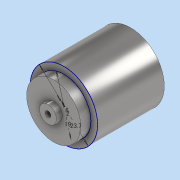
# Autodesk Inventor part: motor_for6speedgearbox
Saved by Autodesk Inventor 2022 (Build 260153000, 153)
## iProperties
Created: 2024-04-30
Part Number: motor_for6speedgearbox
Material: 鉄、可鍛鉄
Document SubType Name: Modeling
Designer: ktamu
Density: 7.15 g/cm^3
Appearance: 半つや出し
Author: ktamu
Autodesk Inventor part; units mm, degrees
ref_plane "YZ Plane" through (0, 0, 0) normal (1, 0, 0) x (0, 1, 0)
ref_plane "XZ Plane" through (0, 0, 0) normal (0, 1, 0) x (-1, 0, 0)
ref_plane "XY Plane" through (0, 0, 0) normal (0, 0, 1) x (1, 0, 0)
sketch "basescetch" plane through (0, 0, 0) normal (0, 0, 1) x (1, 0, 0)
  circle A0 centre (0, 0) radius 11.85
  circle A1 centre (0, 0) radius 9.5
  circle A2 centre (0, 0) radius 3
  circle A3 centre (0, 0) radius 1
  dimension "d0" = 23.7
  dimension "d1" = 19
  dimension "d2" = 6
  dimension "d3" = 2
  constraints: 4 centre point, 4 coincident
  measures "d0" diameter of A0
  measures "d1" diameter of A1
  measures "d2" diameter of A2
  measures "d3" diameter of A3
extrude "押し出し1" add sketch "basescetch" along normal blind 3.5 contours A1
extrude "押し出し2" add sketch "basescetch" along normal blind 5.5 contours A2
extrude "押し出し3" add sketch "basescetch" against normal blind 23.5 contours A0 | A1 | A2 | A3
sketch "スケッチ2" plane through (0, 0, -23.5) normal (0, 0, -1) x (-1, 0, 0)
  circle A0 centre (0, 0) radius 1 projected
  arc A1 (-2, 3.75) -> (2, 3.75) centre (0, 0) ccw
  line L0 (0, -4.25) -> (0, -1)
  line L1 (0, -4.25) -> (8, -4.25) construction
  line L2 (0, 3.75) -> (2, 3.75)
  line L3 (-2, 3.75) -> (0, 3.75)
  dimension "d10" = 8.5
  dimension "d11" = 8
  dimension "d12" = 90
  constraints: 8 end point, 3 point on circle, 1 centre point, 1 coincident, 1 collinear, 1 horizontal, 1 perpendicular, 1 point on line, 1 vertical, 1 vertical alignment, 1 other
  measures "d10" diameter of A1
  measures "d11" distance of L0.start L2.start
  measures "d12" angle of L1 L0
extrude "押し出し4" add sketch "スケッチ2" along normal blind 0.5
extrude "押し出し5" cut sketch "basescetch" against normal through all contours A3
